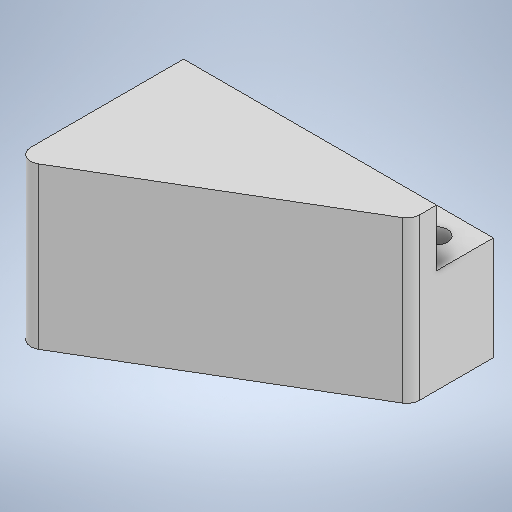
# Autodesk Inventor part: mogo aligner
Saved by Autodesk Inventor 2025.2 (Build 292293000, 293)
## iProperties
Created: 2024-12-10
Part Number: mogo aligner
Material: Generic
Document SubType Name: Modeling
Designer: hmath
Density: 1 g/cm^3
Appearance: Default
Author: hmath
Autodesk Inventor part; units mm, degrees
ref_plane "YZ Plane" through (0, 0, 0) normal (1, 0, 0) x (0, 1, 0)
ref_plane "XZ Plane" through (0, 0, 0) normal (0, 1, 0) x (-1, 0, 0)
ref_plane "XY Plane" through (0, 0, 0) normal (0, 0, 1) x (1, 0, 0)
sketch "Sketch1" plane through (0, 0, 0) normal (0, 0, 1) x (1, 0, 0)
  line L0 (0, 0) -> (52.959, 0)
  line L1 (52.959, 0) -> (52.959, 21.717)
  line L2 (52.959, 21.717) -> (0, 21.717)
  line L3 (0, 21.717) -> (0, 0)
  dimension "d0" = 52.959
  dimension "d1" = 21.717
  constraints: 8 end point, 2 parallel, 1 horizontal, 1 perpendicular
  measures "d0" distance of L1.end L2.end
  measures "d1" distance of L0.end L1.end
extrude "Extrusion1" add sketch "Sketch1" along normal blind 11.9126
sketch "Sketch3" plane through (0, 21.717, 0) normal (0, 1, 0) x (1, 0, 0)
  line L0 (52.959, -11.9126) -> (0, -11.9126) projected
  line L1 (52.959, -11.9126) -> (25.3122, -11.9126)
  line L2 (25.3122, -25.5065) -> (25.3122, -11.9126)
  line L3 (25.3122, -25.5065) -> (25.3122, -33.3756)
  line L4 (52.959, -11.9126) -> (52.959, -16.9926)
  line L5 (52.959, -16.9926) -> (25.3122, -33.3756)
  line L6 (25.3122, -33.3756) -> (25.3122, -34.9664)
  point P0 (0, 0)
  dimension "d20" = 5.08
  dimension "d21" = 21.463
  constraints: 12 end point, 2 vertical, 1 parallel, 1 perpendicular, 1 point on line
  measures "d20" distance of L0.start L4.end
  measures "d21" distance of L3.end L1.end
extrude "Extrusion2" add sketch "Sketch3" against normal up to surface (21.717 mm away)
sketch "Sketch4" plane through (0, 21.717, 0) normal (0, 1, 0) x (1, 0, 0)
  line L0 (52.959, 0) -> (52.959, -16.9926) projected
  line L1 (52.959, 0) -> (52.959, -5.5626)
  line L2 (52.959, -5.5626) -> (46.609, -5.5626)
  circle A0 centre (46.609, -5.5626) radius 2.3241
  line L3 (52.959, 0) -> (0, 0) projected
  circle A1 centre (33.909, -5.5626) radius 2.3241
  circle A2 centre (21.209, -5.5626) radius 2.3241
  circle A3 centre (8.509, -5.5626) radius 2.3241
  circle A4 centre (-4.191, -5.5626) radius 2.3241
  point P0 (52.959, -11.0236)
  dimension "d8" = 6.35
  dimension "d9" = 4.6482
  dimension "d12" = 5.5626
  dimension "d15" = 12.7
  constraints: 5 centre point, 4 end point, 1 coincident, 1 horizontal, 1 perpendicular, 1 point on line, 8 other
  measures "d8" distance of L1.end L2.end
  measures "d9" diameter of A0
  measures "d12" distance between parallel lines of L3 L2
  measures "d15" distance of A0.centre A1.centre
extrude "Extrusion3" cut sketch "Sketch4" against normal through all contours A0 | A1 | A3
sketch "Sketch7" plane through (0, 21.717, 0) normal (0, 1, 0) x (1, 0, 0)
  line L0 (52.959, 0) -> (52.959, -16.9926) projected
  line L1 (25.3122, -33.3756) -> (52.959, -16.9926) projected
  line L2 (52.959, -16.9926) -> (25.3122, -33.3756)
  line L3 (25.3122, -33.3756) -> (0, -48.3751)
  line L4 (0, 0) -> (0, -11.9126) projected
  line L5 (0, -48.3751) -> (0, -11.9126)
  line L6 (0, -11.9126) -> (25.3122, -11.9126)
  line L7 (25.3122, -11.9126) -> (52.959, -11.9126)
  line L8 (52.959, -11.9126) -> (52.959, -16.9926)
  constraints: 12 end point, 2 collinear, 2 perpendicular, 2 point on line
extrude "Extrusion5" add sketch "Sketch7" along normal blind 11.9126
sketch "Sketch8" plane through (0, 21.717, 0) normal (0, -1, 0) x (1, 0, 0)
  line L0 (0, 48.3751) -> (52.959, 16.9926) projected
  line L1 (0, 11.9126) -> (25.3122, 11.9126) projected
  line L2 (0, 48.3751) -> (0, 11.9126)
  line L3 (25.3122, 11.9126) -> (52.959, 11.9126) projected
  line L4 (0, 11.9126) -> (25.3122, 11.9126)
  line L5 (25.3122, 11.9126) -> (25.3122, 33.3756) projected
  line L6 (25.3122, 11.9126) -> (25.3122, 33.3756)
  line L7 (0, 48.3751) -> (25.3122, 33.3756) projected
  line L8 (25.3122, 33.3756) -> (0, 48.3751)
  point P0 (0, 0)
  constraints: 8 end point, 2 collinear, 1 perpendicular, 1 vertical
extrude "Extrusion6" add sketch "Sketch8" along normal up to surface (21.717 mm away)
fillet "Fillet6" radius 2.54 2 edges at (52.959, 16.8148, 16.9926) (0, 16.8148, 48.3751)
sketch "Sketch9" plane through (0, 0, 0) normal (0, 0, -1) x (-1, 0, 0)
  line L0 (0, 21.717) -> (-8.509, 21.717)
  line L1 (-10.8331, 21.717) -> (-6.1849, 21.717) projected
  line L2 (-8.509, 21.717) -> (-8.509, 16.383)
  circle A0 centre (-8.509, 16.383) radius 2.3241
  point P0 (0, 0)
  dimension "d32" = 8.509
  dimension "d33" = 5.334
  dimension "d34" = 4.6482
  constraints: 4 end point, 1 centre point, 1 coincident, 1 midpoint, 1 perpendicular
  measures "d32" distance of L0.start L0.end
  measures "d33" distance of L0.end L2.end
  measures "d34" diameter of A0
extrude "Extrusion7" cut sketch "Sketch9" against normal blind 6.35
body "Solid1"
